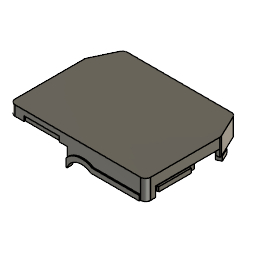
logger_case_top (Autodesk Fusion 360 design; units mm, degrees)
part number: 2026-07-28-15-39-10-623
Autodesk Fusion 360 part; units mm, degrees
sketch "Skizze1" plane through (0, 0, 0) normal (0, 0, 1) x (1, 0, 0)
  line L0 (0, 0) -> (-54, 0)
  line L1 (-54, 0) -> (-54, 30)
  line L2 (-54, 30) -> (-49, 40.5)
  line L3 (-49, 40.5) -> (-5, 40.5)
  line L4 (-5, 40.5) -> (0, 30)
  line L5 (0, 30) -> (0, 0)
  dimension "d1" = 54
  dimension "d2" = 30
  dimension "d3" = 10.5
  dimension "d4" = 44
  dimension "d5" = 5
  dimension "d6" = 5
  dimension "d7" = 30
  dimension "d8" = 10.5
  dimension "d9" = 40.5
  constraint coincident L0.start L5.end
  constraint horizontal L0
  constraint perpendicular L0 L1
  constraint perpendicular L1 L3
  constraint perpendicular L0 L5
  measures "d1" distance of L0.start L0.end
  measures "d2" distance of L0.start L4.end
  measures "d3" distance of L3 L4.end
  measures "d4" distance of L2.end L3.end
  measures "d5" horizontal distance of L3.end L4.end
  measures "d6" horizontal distance of L1.end L2.end
  measures "d7" distance of L0.end L1.end
  measures "d8" vertical distance of L1.end L2.end
  measures "d9" distance of L0 L3
extrude "Extrusion1" add sketch "Skizze1" against normal blind 2 makes body 1
fillet "Abrundung1" radius 2 1 edges at (0, 30, -1) on bodies 1
fillet "Abrundung2" radius 2 1 edges at (0, 0, -1) on bodies 1
fillet "Abrundung3" radius 2 1 edges at (-5, 40.5, -1) on bodies 1
fillet "Abrundung4" radius 2 1 edges at (-49, 40.5, -1) on bodies 1
fillet "Abrundung5" radius 2 1 edges at (-54, 30, -1) on bodies 1
fillet "Abrundung6" radius 2 1 edges at (-54, 0, -1) on bodies 1
sketch "Skizze2" plane through (0, 0, -2) normal (0, 0, -1) x (1, 0, 0)
  line L0 (-4.4571, -39.3599) -> (-0.1943, -30.408)
  line L1 (0, -29.5481) -> (0, -2)
  line L2 (-2, 0) -> (-52, 0)
  line L3 (-54, -2) -> (-54, -29.5481)
  line L4 (-53.8057, -30.408) -> (-49.5429, -39.3599)
  line L5 (-47.7372, -40.5) -> (-6.2628, -40.5)
  line L6 (-2, 0) -> (-52, 0)
  line L7 (0, -29.5481) -> (0, -2)
  line L8 (-4.4571, -39.3599) -> (-0.1943, -30.408)
  line L9 (-47.7372, -40.5) -> (-6.2628, -40.5)
  line L10 (-53.8057, -30.408) -> (-49.5429, -39.3599)
  line L11 (-54, -2) -> (-54, -29.5481)
  arc A0 (-52, 0) -> (-54, -2) centre (-52, -2) ccw
  arc A1 (-54, -29.5481) -> (-53.8057, -30.408) centre (-52, -29.5481) ccw
  arc A2 (-49.5429, -39.3599) -> (-47.7372, -40.5) centre (-47.7372, -38.5) ccw
  arc A3 (-6.2628, -40.5) -> (-4.4571, -39.3599) centre (-6.2628, -38.5) ccw
  arc A4 (-0.1943, -30.408) -> (0, -29.5481) centre (-2, -29.5481) ccw
  arc A5 (0, -2) -> (-2, 0) centre (-2, -2) ccw
  line L12 (-52.3611, -29.7201) -> (-48.0983, -38.672)
  arc A6 (-48.0983, -38.672) -> (-47.7372, -38.9) centre (-47.7372, -38.5) ccw
  line L13 (-47.7372, -38.9) -> (-6.2628, -38.9)
  arc A7 (-6.2628, -38.9) -> (-5.9017, -38.672) centre (-6.2628, -38.5) ccw
  line L14 (-5.9017, -38.672) -> (-1.6389, -29.7201)
  arc A8 (-1.6389, -29.7201) -> (-1.6, -29.5481) centre (-2, -29.5481) ccw
  line L15 (-1.6, -29.5481) -> (-1.6, -2)
  arc A9 (-1.6, -2) -> (-2, -1.6) centre (-2, -2) ccw
  line L16 (-2, -1.6) -> (-52, -1.6)
  arc A10 (-52, -1.6) -> (-52.4, -2) centre (-52, -2) ccw
  line L17 (-52.4, -2) -> (-52.4, -29.5481)
  arc A11 (-52.4, -29.5481) -> (-52.3611, -29.7201) centre (-52, -29.5481) ccw
  dimension "d12" = -1.6
extrude "Extrusion2" add sketch "Skizze2" along normal blind 9 separate body makes body 2
sketch "Skizze3" plane through (0, 0, 0) normal (0, -1, 0) x (1, 0, 0)
  line L0 (-52, -11) -> (-2, -11)
  line L1 (-52, -11) -> (-31.4, -11)
  line L2 (-18.7578, -11) -> (-20, -11)
  line L3 (-54, -2) -> (-54, -11) construction
  line L4 (0, -2) -> (0, -11) construction
  line L5 (0, -8) -> (0, -11)
  line L6 (0, -11) -> (-18.7578, -11)
  circle A0 centre (-25, -13) radius 6.2
  line L7 (0, -8) -> (-21.3339, -8)
  line L8 (-2, -2) -> (-52, -2)
  line L9 (-54, -11) -> (-54, -4)
  line L10 (-31.2, -4) -> (-31.2, -11)
  line L11 (-31.2, -4) -> (-54, -4)
  line L12 (-54, -11) -> (-31.2, -11)
  dimension "d140" = 12.4
  dimension "d142" = 25
  dimension "d145" = 2
  dimension "d146" = 22.8
  dimension "d155" = 11
  dimension "d156" = 6
  dimension "d157" = 3
  constraint coincident L0 L1.end
  constraint coincident L0.start L1.start
  constraint horizontal L2
  constraint coincident L0 L2.start
  constraint coincident L4 L5.start
  constraint coincident L4.end L5.end
  constraint coincident A0 L7.end
  constraint perpendicular L5 L7
  constraint coincident L3.end L9.start
  constraint coincident L3 L9.end
  constraint coincident L1 L10.end
  constraint perpendicular L9 L11
  measures "d140" diameter of A0
  measures "d142" distance of L5 A0.centre
  measures "d145" distance of L8 L11
  measures "d146" distance of L9 L10
  measures "d155" distance of A0.centre L8
  measures "d156" distance of L7 L8
  measures "d157" distance of L5.start L4.end
extrude "Extrusion23" cut sketch "Skizze3" against normal blind 2 contours L0 L2 A0 | L0 L2 A0 bodies 2
extrude "Extrusion24" cut sketch "Skizze3" against normal blind 4 contours L0 L2 L5 L6 A0 L7 bodies 2
extrude "Extrusion3" cut sketch "Skizze3" against normal blind 2 contours L0 L1 L9 L10 L11 L12 bodies 2
sketch "Skizze4" plane through (0, 0, 0) normal (0, -1, 0) x (1, 0, 0)
  line L0 (-48.4, -4) -> (-48.4, -2)
  line L1 (-52, -2) -> (-52, -4)
  line L2 (-48.4, -2) -> (-34.4, -2)
  line L3 (-34.4, -2) -> (-34.4, -4)
  line L4 (-34.4, -4) -> (-48.4, -4)
  line L5 (-54, -2) -> (-54, -4)
  line L6 (-31.2, -4) -> (-31.2, -11)
  dimension "d48" = 14
  dimension "d50" = 2
  dimension "d51" = 2
  dimension "d66" = 5.6
  dimension "d151" = 3.2
  constraint vertical L0
  constraint perpendicular L0 L2
  constraint perpendicular L2 L3
  measures "d48" distance of L0.end L2.end
  measures "d50" distance of L2.end L3.end
  measures "d51" distance of L0.start L0.end
  measures "d66" distance of L0 L5
  measures "d151" distance of L3 L6
extrude "Extrusion7" cut sketch "Skizze4" against normal blind 0.5 bodies 2
sketch "Skizze5" plane through (0, 0, 0) normal (0, -1, 0) x (1, 0, 0)
  line L0 (-21.3339, -8) -> (-2, -8)
  line L1 (-2, -6) -> (-2, -8)
  line L2 (-31.2, -11) -> (-31.2, -5.6334)
  line L3 (-31.2, -11) -> (-30.8686, -11)
  arc A0 (-21.3339, -8) -> (-30.8686, -11) centre (-25, -13) ccw
  line L4 (-20.7292, -6) -> (-2, -6)
  arc A1 (-20.7292, -6) -> (-32.7616, -10.3548) centre (-25, -13) ccw
  dimension "d158" = 2
  constraint coincident L0.end L1.end
  constraint perpendicular L0 L1
extrude "Extrusion25" add sketch "Skizze5" along normal blind 0.5 bodies 2
sketch "Skizze6" plane through (-54, 0, 0) normal (-1, 0, 0) x (0, -1, 0)
  line L0 (-2, -2) -> (-29.5481, -2)
  line L1 (-29.5481, -2) -> (-29.5481, -11)
  line L2 (-29.5481, -11) -> (-2, -11)
  line L3 (-29.5481, -11) -> (0, -11)
  line L4 (-2, 0) -> (-29.5481, 0) construction
  line L5 (-29.5481, -11) -> (-29.5481, -4)
  line L6 (0, -4) -> (-29.5481, -4)
  line L7 (0, -4) -> (0, -11)
  line L8 (-2, -11) -> (-2, -4)
  dimension "d61" = 4
  constraint coincident L1.end L2.start
  constraint coincident L1 L5.end
  constraint perpendicular L5 L6
  constraint perpendicular L3 L7
  measures "d61" distance of L4 L6
extrude "Extrusion10" cut sketch "Skizze6" against normal blind 2 bodies 2
sketch "Skizze8" plane through (0, 40.5, 0) normal (0, 1, 0) x (-1, 0, 0)
  line L0 (47.7372, -2) -> (6.2628, -2)
  line L1 (6.2628, -2) -> (6.2628, -11)
  line L2 (6.2628, -11) -> (47.7372, -11)
  line L3 (61.5002, -11) -> (61.5002, -7)
  line L4 (47.7372, 0) -> (6.2628, 0)
  line L5 (61.5002, -7) -> (37.5143, -7)
  line L6 (37.5143, -7) -> (37.5143, -11)
  line L7 (61.5002, -11) -> (37.5143, -11)
  dimension "d81" = 5
  constraint perpendicular L2 L3
  constraint perpendicular L3 L5
  constraint coincident L2 L6.end
  constraint perpendicular L2 L6
  constraint horizontal L7
  measures "d81" distance of L0 L5
extrude "Extrusion11" cut sketch "Skizze8" against normal blind 15 bodies 2
sketch "Skizze9" plane through (0, 40.5, 0) normal (0, 1, 0) x (-1, 0, 0)
  line L0 (47.7372, -2) -> (6.2628, -2)
  line L1 (6.2628, -2) -> (6.2628, -11)
  line L2 (6.2628, -11) -> (37.5143, -11)
  line L3 (47.7372, -7) -> (47.7372, -2)
  line L4 (9.4998, -11) -> (9.4998, -4)
  line L5 (9.4998, -4) -> (44.4998, -4)
  line L6 (44.4998, -4) -> (44.4998, -11)
  line L7 (44.4998, -11) -> (9.4998, -11)
  line L8 (47.7372, 0) -> (6.2628, 0)
  line L9 (37.5143, -7) -> (47.7372, -7)
  line L10 (37.5143, -11) -> (37.5143, -7)
  dimension "d72" = 4
  dimension "d73" = 35
  dimension "d75" = 3.237
  constraint coincident L2 L4.start
  constraint perpendicular L2 L4
  constraint perpendicular L4 L5
  constraint coincident L2 L6.end
  constraint perpendicular L2 L6
  measures "d72" distance of L5 L8
  measures "d73" distance of L4.end L5.end
  measures "d75" distance of L1 L4
extrude "Extrusion12" cut sketch "Skizze9" against normal blind 2 contours L2 L4 L5 L6 L7 L9 L10 | L6 L7 L9 L10 bodies 2
sketch "Skizze11" plane through (0, 0, 0) normal (1, 0, 0) x (0, 1, 0)
  line L0 (2, -2) -> (2, -8)
  line L1 (4, -11) -> (29.5481, -11)
  line L2 (29.5481, -11) -> (29.5481, -2)
  line L3 (2, -4) -> (29.5481, -4)
  line L4 (29.5481, 0) -> (2, 0)
  line L5 (4, -8) -> (4, -11)
  line L6 (4, -8) -> (4, -4)
  dimension "d84" = 4
  constraint coincident L0 L3.start
  constraint coincident L2 L3.end
  constraint perpendicular L2 L3
  constraint coincident L5.start L6.start
  constraint coincident L3 L6.end
  constraint perpendicular L3 L6
  measures "d84" distance of L3 L4
extrude "Extrusion13" cut sketch "Skizze11" against normal blind 2 bodies 2
sketch "Skizze10" plane through (0, 40.5, 0) normal (0, 1, 0) x (-1, 0, 0)
  line L0 (9.4998, -4) -> (44.4998, -4)
  line L1 (44.4998, -4) -> (44.4998, -7)
  line L2 (44.4998, -7) -> (47.7372, -7)
  line L3 (47.7372, -7) -> (47.7372, -2)
  line L4 (47.7372, -2) -> (6.2628, -2)
  line L5 (6.2628, -11) -> (9.4998, -11)
  line L6 (-2, -7) -> (11, -7)
  line L7 (11, -7) -> (11, -15)
  line L8 (11, -15) -> (-2, -15)
  line L9 (-2, -15) -> (-2, -7)
  line L10 (47.7372, 0) -> (6.2628, 0)
  dimension "d82" = 7
  constraint perpendicular L6 L7
  constraint perpendicular L6 L9
  measures "d82" distance of L6 L10
extrude "Extrusion14" cut sketch "Skizze10" against normal blind 15 bodies 2
sketch "Skizze13" plane through (-52.4, 0, 0) normal (1, 0, 0) x (0, 1, 0)
  line L0 (29.5481, -4) -> (29.5481, -2)
  line L1 (29.5481, -2) -> (2, -2)
  line L2 (2, -2) -> (2, -4)
  line L3 (4, -2) -> (4, -7.5)
  line L4 (4, -7.5) -> (21, -7.5)
  line L5 (21, -7.5) -> (21, -2)
  dimension "d89" = 5.5
  dimension "d91" = 2
  dimension "d93" = 17
  constraint coincident L1 L3.start
  constraint perpendicular L1 L3
  constraint perpendicular L3 L4
  constraint coincident L1 L5.end
  constraint perpendicular L1 L5
  measures "d89" distance of L1 L4
  measures "d91" distance of L2 L3
  measures "d93" distance of L3.end L4.end
extrude "Extrusion15" add sketch "Skizze13" along normal blind 1.3 separate body makes body 3
sketch "Skizze14" plane through (-52.4, 0, 0) normal (-1, 0, 0) x (0, -1, 0)
  line L0 (-21, -2) -> (-21, -7.5)
  line L1 (-21, -7.5) -> (-4, -7.5)
  line L2 (-4, -7.5) -> (-4, -2)
  line L3 (-4, -2) -> (-21, -2)
  line L4 (-19, -7.5) -> (-19, -5.7)
  line L5 (-19, -5.7) -> (-6, -5.7)
  line L6 (-19, -7.5) -> (-6, -7.5)
  line L7 (-6, -5.7) -> (-6, -7.5)
  line L8 (-2, -4) -> (-29.5481, -4)
  dimension "d96" = 1.8
  dimension "d97" = 1.7
  dimension "d98" = 2
  dimension "d99" = 2
  dimension "d120" = 13
  constraint coincident L1 L4.start
  constraint perpendicular L1 L4
  constraint perpendicular L4 L5
  constraint coincident L1 L6.end
  constraint parallel L4 L7
  measures "d96" distance of L4.start L4.end
  measures "d97" distance of L5 L8
  measures "d98" distance of L0 L4
  measures "d99" distance of L2 L7
  measures "d120" distance of L4.end L5.end
extrude "Extrusion16" add sketch "Skizze14" along normal blind 0.8 contours L1 L4 L5 L6 L7 bodies 3
sketch "Skizze15" plane through (-54.219, 25.8186, 0) normal (0.902861, -0.429934, 0) x (0.429934, 0.902861, 0)
  line L0 (14.2363, -7) -> (14.2363, -2)
  line L1 (14.2363, -2) -> (4.3213, -2)
  line L2 (4.3213, -2) -> (4.3213, -7)
  line L3 (7.3213, -2) -> (7.3213, -11)
  line L4 (7.3213, -11) -> (11.3213, -11)
  line L5 (11.3213, -11) -> (11.3213, -2)
  line L6 (7.3213, -2) -> (11.3213, -2)
  dimension "d102" = 9
  dimension "d103" = 3
  dimension "d105" = 4
  dimension "d106" = 2.915
  dimension "d109" = 4
  constraint coincident L1 L3.start
  constraint perpendicular L3 L4
  constraint coincident L1 L5.end
  constraint perpendicular L1 L5
  measures "d102" distance of L3.start L3.end
  measures "d103" distance of L2 L3
  measures "d105" distance of L3.end L4.end
  measures "d106" distance of L0 L5
  measures "d109" distance of L0.start L4
extrude "Extrusion17" add sketch "Skizze15" along normal blind 1.3 separate body makes body 4
sketch "Skizze16" plane through (-54.219, 25.8186, 0) normal (-0.902861, 0.429934, 0) x (-0.429934, -0.902861, 0)
  line L0 (-11.3213, -11) -> (-7.3213, -11)
  line L1 (-7.3213, -11) -> (-7.3213, -2)
  line L2 (-7.3213, -2) -> (-11.3213, -2)
  line L3 (-11.3213, -2) -> (-11.3213, -11)
  line L4 (-11.3213, -9.2) -> (-11.3213, -11)
  line L5 (-7.3213, -11) -> (-7.3213, -9.2)
  line L6 (-11.3213, -9.2) -> (-7.3213, -9.2)
  line L7 (22.5508, -2) -> (21.4107, -2)
  line L8 (21.4107, -2) -> (-3.4614, -2)
  line L9 (-3.4614, -2) -> (-4.3213, -2)
  line L10 (-4.3213, -2) -> (-14.2363, -2)
  line L11 (-14.2363, -2) -> (-16.042, -2)
  line L12 (-16.042, -2) -> (-33.8733, -2)
  line L13 (-33.6202, -2) -> (-34.0675, -2)
  line L14 (-33.6202, -2) -> (-27.3706, -2)
  line L15 (-26.6778, -2) -> (-27.3706, -2)
  line L16 (-26.6778, -2) -> (-1.8057, -2)
  line L17 (0.8599, -2) -> (-1.8057, -2)
  line L18 (0.8599, -2) -> (22.3565, -2)
  dimension "d110" = 1.8
  dimension "d111" = 4
  constraint coincident L3 L4.start
  constraint coincident L0.start L3.end
  constraint coincident L0.end L1.start
  constraint coincident L1 L5.end
  constraint horizontal L6
  measures "d110" distance of L0.end L5.end
  measures "d111" distance of L4 L5
extrude "Extrusion18" add sketch "Skizze16" along normal blind 0.8 contours L0 L1 L3 L4 L5 L6 bodies 4
sketch "Skizze17" plane through (-1.6, 0, 0) normal (-1, 0, 0) x (0, -1, 0)
  line L0 (-2, -8) -> (-2, -2)
  line L1 (-2, -2) -> (-29.5481, -2)
  line L2 (-29.5481, -2) -> (-29.5481, -4)
  line L3 (-21, -2) -> (-21, -7.5)
  line L4 (-21, -7.5) -> (-4, -7.5)
  line L5 (-4, -7.5) -> (-4, -2)
  line L6 (-4, -4) -> (-4, -8)
  line L7 (-4, -8) -> (-2, -8)
  dimension "d114" = 17
  dimension "d115" = 2
  dimension "d116" = 8.5481
  dimension "d117" = 5.5
  constraint coincident L1 L3.start
  constraint perpendicular L3 L4
  constraint coincident L1 L5.end
  constraint perpendicular L1 L5
  measures "d114" distance of L3.end L4.end
  measures "d115" distance of L0 L5
  measures "d116" distance of L2 L3
  measures "d117" distance of L1 L4
extrude "Extrusion19" add sketch "Skizze17" along normal blind 1.3 contours L1 L3 L4 L5 L6 bodies 1 3 4 2
sketch "Skizze18" plane through (-1.6, 0, 0) normal (1, 0, 0) x (0, 1, 0)
  line L0 (21, -4) -> (4, -4)
  line L1 (4, -7.5) -> (21, -7.5)
  line L2 (21, -7.5) -> (21, -4)
  line L3 (6, -5.7) -> (6, -7.5)
  line L4 (6, -7.5) -> (19, -7.5)
  line L5 (19, -7.5) -> (19, -5.7)
  line L6 (19, -5.7) -> (6, -5.7)
  line L7 (4, -4) -> (4, -7.5)
  dimension "d122" = 2
  dimension "d123" = 13
  dimension "d125" = 1.7
  constraint coincident L1 L3.end
  constraint perpendicular L1 L3
  constraint coincident L1 L4.end
  constraint perpendicular L4 L5
  constraint parallel L4 L6
  measures "d122" distance of L2 L5
  measures "d123" horizontal distance of L3.start L5.end
  measures "d125" distance of L0 L6
extrude "Extrusion20" add sketch "Skizze18" along normal blind 0.8 contours L1 L3 L4 L5 L6 bodies 1
sketch "Skizze19" plane through (10.2005, 4.8574, 0) normal (-0.902861, -0.429934, 0) x (0.429934, -0.902861, 0)
  line L0 (-27.5377, -7) -> (-27.5377, -2)
  line L1 (-27.5377, -2) -> (-37.4527, -2)
  line L2 (-37.4527, -2) -> (-37.4527, -7)
  line L3 (-34.5377, -2) -> (-34.5377, -11)
  line L4 (-34.5377, -11) -> (-30.5377, -11)
  line L5 (-30.5377, -11) -> (-30.5377, -2)
  dimension "d128" = 9
  dimension "d129" = 4
  dimension "d130" = 3
  dimension "d131" = 2.915
  constraint coincident L1 L3.start
  constraint perpendicular L1 L3
  constraint perpendicular L3 L4
  constraint coincident L1 L5.end
  constraint perpendicular L1 L5
  measures "d128" distance of L4.end L5.end
  measures "d129" distance of L3.end L4.end
  measures "d130" distance of L0 L5
  measures "d131" distance of L2 L3
extrude "Extrusion21" add sketch "Skizze19" along normal blind 1.3 bodies 1
sketch "Skizze20" plane through (10.2005, 4.8574, 0) normal (0.902861, 0.429934, 0) x (-0.429934, 0.902861, 0)
  line L0 (34.5377, -7) -> (30.5377, -7)
  line L1 (30.5377, -7) -> (30.5377, -11)
  line L2 (30.5377, -11) -> (34.5377, -11)
  line L3 (34.5377, -11) -> (34.5377, -7)
  line L4 (30.5377, -11) -> (30.5377, -9.2)
  line L5 (30.5377, -9.2) -> (34.5377, -9.2)
  line L6 (34.5377, -9.2) -> (34.5377, -11)
  dimension "d134" = 4
  dimension "d135" = 1.8
  constraint coincident L1.end L2.start
  constraint coincident L1 L4.end
  constraint coincident L3 L5.end
  constraint perpendicular L3 L5
  constraint coincident L2.end L3.start
  measures "d134" distance of L1.end L2.end
  measures "d135" distance of L5.end L2.end
extrude "Extrusion22" add sketch "Skizze20" along normal blind 0.8 contours L1 L2 L3 L4 L5 L6 bodies 1
